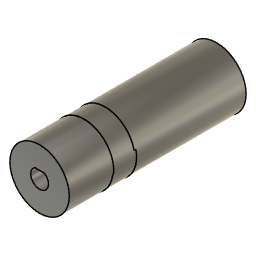
shaft_model (Autodesk Fusion 360 design; units mm, degrees)
Autodesk Fusion 360 part; units mm, degrees
sketch "Sketch1" plane through (0, 0, 0) normal (0, 0, 1) x (1, 0, 0)
  line L0 (0, 2.5112) -> (1.6437, 2.5096)
  line L1 (-1.6437, 2.5096) -> (0, 2.5112)
  arc A0 (-1.6437, 2.5096) -> (1.6437, 2.5096) centre (0, 0) ccw
  circle A1 centre (0, 0) radius 7.5
  line L2 (16.998, 0.0035) -> (18.7305, -2.9961)
  line L3 (18.7305, -2.9961) -> (22.1945, -2.9961)
  line L4 (22.1945, -2.9961) -> (23.9337, -0.0004)
  line L5 (23.9337, -0.0004) -> (22.2095, 3.0041)
  line L6 (22.2095, 3.0041) -> (18.7455, 3.0041)
  line L7 (18.7455, 3.0041) -> (16.998, 0.0035)
  circle A2 centre (20.4658, 0.0016) radius 7.5
  dimension "d1" = 6
  dimension "d3" = 15
  dimension "d4" = 3.464
  dimension "d5" = 3.464
  dimension "d6" = 3.464
  dimension "d7" = 3.464
  dimension "d8" = 3.464
  dimension "d9" = 15
  constraint coincident A0.centre A1.centre
  constraint horizontal L3
  constraint parallel L3 L6
  measures "d1" diameter of A0
  measures "d3" diameter of A1
  measures "d4" distance of L2.start L2.end
  measures "d5" distance of L2.end L3.end
  measures "d6" distance of L3.end L4.end
  measures "d7" distance of L4.end L5.end
  measures "d8" distance of L5.end L6.end
  measures "d9" diameter of A2
extrude "Extrude1" add sketch "Sketch1" along normal blind 15 makes body 1 at (7.4627, -0.7468, 10) makes body 2 at (27.9286, -0.7452, 10)
move_face "OffsetFaces1" offset 20 1 faces at (16.6708, 2.4113, 0) on bodies 2
sketch "Sketch2" plane through (0, 0, 0) normal (1, 0, 0) x (0, 1, 0)
sketch "Sketch3" plane through (0, 0, 0) normal (0, 0, 1) x (1, 0, 0)
  circle A0 centre (-35, 0) radius 10
  dimension "d14" = 20
  measures "d14" diameter of A0
extrude "Extrude2" add sketch "Sketch3" along normal blind 8 separate body makes body 3
move_face "OffsetFaces2" offset 2.5 1 faces at (7.4627, -0.7468, 10) on bodies 1
move_body "Move1" bodies 1 to x (1, 0, 0) y (0, 1, 0) z (0, 0, 1) at (-12.879, -0.6739, 0)
move_face "OffsetFaces3" offset 2.5 2 faces at (27.9565, 0.3754, -8.3333) (16.6708, 2.4113, 15) on bodies 2
sketch "Sketch4" plane through (0, 0, 0) normal (0, 1, 0) x (1, 0, 0)
move_body "Move2" bodies 1 to x (1, 0, 0) y (0, 1, 0) z (0, 0, 1) at (33.2972, 0.686, 18.7517)
sketch "Sketch5" plane through (0, 0, 0) normal (0, 1, 0) x (1, 0, 0)
move_body "Move3" bodies 2 to x (1, 0, 0) y (0, 1, 0) z (0, 0, 1) at (-10.4244, 0, -1.9102)
move_face "MoveFace1" to x (1, 0, 0) y (0, 1, 0) z (0, 0, 1) at (-0.0251, 0, -0.2139) 1 faces at (20.029, 0.5, 3.0898) on bodies 2
move_body "Move4" bodies 1 to x (1, 0, 0) y (0, 1, 0) z (0, 0, 1) at (-10.3871, 0, 3.9543)
move_face "MoveFace2" to x (0.996195, -0.087156, 0) y (0.087156, 0.996195, 0) z (0, 0, 1) at (22.3045, -3.8796, 17.9955) 1 faces at (-25.0124, -0.4985, 5.3333) on bodies 3
move_body "Move5" bodies 3 to x (1, 0, 0) y (0, 1, 0) z (0, 0, 1) at (22, 0, 15)
move_face "MoveFace3" to x (1, 0, 0) y (0, 1, 0) z (0, 0, 1) at (0.5878, 0.7902, 1.2243) 1 faces at (19.3438, -2.1961, 20.3333) on bodies 3
combine "Combine1" operation add target body 3 tool bodies 1
combine "Combine2" operation add target body 2 tool bodies 3
move_body "Move6" bodies 2 to x (1, 0, 0) y (0, 0, 1) z (0, -1, 0) at (0, -31.9491, -11.8713)
